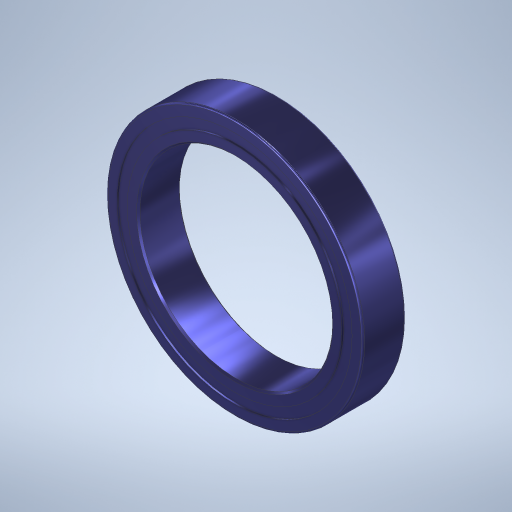
# Autodesk Inventor part: Front Hub Bearing
Saved by Autodesk Inventor 2023.1 (Build 271208000, 208)
## iProperties
Created: 2019-11-25
Part Number: Front Hub Bearing
Material: Generic
Document SubType Name: Modeling
Designer: Jopa
Density: 1 g/cm^3
Appearance: Poplar
Author: Jopa
Autodesk Inventor part; units mm, degrees
ref_plane "YZ Plane" through (0, 0, 0) normal (1, 0, 0) x (0, 1, 0)
ref_plane "XZ Plane" through (0, 0, 0) normal (0, 1, 0) x (-1, 0, 0)
ref_plane "XY Plane" through (0, 0, 0) normal (0, 0, 1) x (1, 0, 0)
sketch "Sketch1" plane through (0, 0, 0) normal (0, 0, 1) x (1, 0, 0)
  circle A0 centre (0, 0) radius 7.1437
  circle A1 centre (0, 0) radius 7.9566
  circle A2 centre (0, 0) radius 9.525
  circle A3 centre (0, 0) radius 8.7122
  dimension "d0" = 14.2875
  dimension "d1" = 0.8128
  dimension "d2" = 19.05
  dimension "d3" = 0.8128
  constraints: 4 centre point, 2 coincident
  measures "d0" diameter of A0
  measures "d1" radial gap between concentric circles of A0 A1
  measures "d2" diameter of A2
  measures "d3" radial gap between concentric circles of A2 A3
extrude "Extrusion1" add sketch "Sketch1" along normal mid plane 3.175
fillet "Fillet1" radius 0.127 2 edges at (-9.525, 0, 1.5875) (-9.525, 0, -1.5875)
chamfer "Chamfer1" distance 0.127 angle 45 2 edges at (-7.1437, 0, 1.5875) (-7.1437, 0, -1.5875)
extrude "Extrusion2" add sketch "Sketch1" along normal mid plane 2.921 contours A3
body "Solid1"
